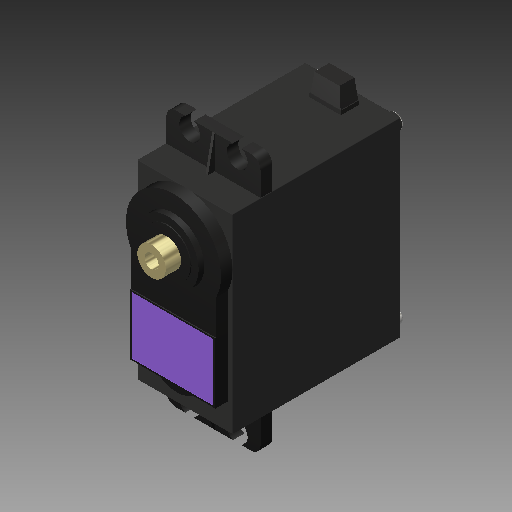
# Autodesk Inventor part: Servomotor
Saved by Autodesk Inventor 2017 (Build 210142000, 142)
## iProperties
Created: 2019-10-22
Part Number: Servomotor
Material: Generic
Document SubType Name: Modeling
Designer: User
Density: 1 g/cm^3
Appearance: Glossy - Black
Mass: 31.6887 g
Surface Area: 70.3531 cm^2
Volume: 31.6887 cm^3
Author: User
Autodesk Inventor part; units mm, degrees
ref_plane "YZ Plane" through (0, 0, 0) normal (1, 0, 0) x (0, 1, 0)
ref_plane "XZ Plane" through (0, 0, 0) normal (0, 1, 0) x (-1, 0, 0)
ref_plane "XY Plane" through (0, 0, 0) normal (0, 0, 1) x (1, 0, 0)
sketch "Sketch1" plane through (0, 0, 0) normal (0, 0, 1) x (1, 0, 0)
  line L0 (-10, 20) -> (10, 20)
  line L1 (10, 20) -> (10, -20)
  line L2 (10, -20) -> (-10, -20)
  line L3 (-10, -20) -> (-10, 20)
  line L4 (-10, 20) -> (10, -20) construction
  line L5 (10, 20) -> (-10, -20) construction
  point P0 (0, 0)
  dimension "d0" = 20
  dimension "d1" = 40
  constraints: 12 end point, 2 midpoint, 2 parallel, 1 horizontal, 1 perpendicular
  measures "d0" distance of L1.end L2.end
  measures "d1" distance of L0.end L1.end
extrude "Extrusion1" add sketch "Sketch1" along normal blind 36.88
chamfer "Chamfer1" distance 1.64 angle 45 4 edges at (-10, 0, 0) (0, 20, 0) (10, 0, 0) (0, -20, 0)
ref_plane "Work Plane1" through (0, 0, 1) normal (0, 0, -1) x (-1, 0, 0)
sketch "Sketch2" plane through (0, 0, 1) normal (0, 0, -1) x (-1, 0, 0)
  line L0 (9.36, -19.36) -> (-9.36, -19.36) projected
  line L1 (-9.36, -19.36) -> (-9.36, 19.36) projected
  line L2 (-9.36, 19.36) -> (9.36, 19.36) projected
  line L3 (9.36, 19.36) -> (9.36, -19.36) projected
  arc A0 (9.36, -15.36) -> (5.36, -19.36) centre (9.36, -19.36) ccw
  point P0 (0, 0)
  dimension "d8" = 8
  constraints: 2 point on circle, 2 point on line, 1 centre point, 1 coincident
  measures "d8" diameter of A0
extrude "Extrusion2" cut sketch "Sketch2" along normal up to next contours L0 A0 L3
mirror "Mirror1" about plane through (0, 0, 0) normal (0, 1, 0) of "Extrusion2"
mirror "Mirror2" about plane through (0, 0, 0) normal (1, 0, 0) of "Extrusion2", "Mirror1"
sketch "Sketch3" plane through (9.36, 19.36, 1) normal (0, 0, -1) x (-1, 0, 0)
  arc A0 (4, -38.72) -> (0, -34.72) centre (0, -38.72) ccw projected
  line L0 (0, -38.72) -> (0, -34.72) projected
  line L1 (4, -38.72) -> (0, -38.72) projected
  line L2 (14.72, -38.72) -> (4, -38.72) projected
  arc A1 (18.72, -34.72) -> (14.72, -38.72) centre (18.72, -38.72) ccw projected
  line L3 (18.72, -4) -> (18.72, -34.72) projected
  arc A2 (14.72, 0) -> (18.72, -4) centre (18.72, 0) ccw projected
  line L4 (4, 0) -> (14.72, 0) projected
  arc A3 (0, -4) -> (4, 0) centre (0, 0) ccw projected
  line L5 (0, -4) -> (0, 0) projected
  line L6 (0, 0) -> (4, 0) projected
  line L7 (0, -34.72) -> (0, -4) projected
  line L8 (18.72, -38.72) -> (14.72, -38.72) projected
  line L9 (18.72, -34.72) -> (18.72, -38.72) projected
  line L10 (18.72, 0) -> (18.72, -4) projected
  line L11 (14.72, 0) -> (18.72, 0) projected
  line L12 (0, -4) -> (0, 0) projected
  line L13 (0, 0) -> (1.6569, 0) construction
  circle A4 centre (1.6569, -1.6569) radius 1.6
  point P0 (9.36, -19.36)
  dimension "d16" = 3.2
  constraints: 2 end point, 1 centre point, 1 horizontal, 1 point on circle
  measures "d16" diameter of A4
extrude "Extrusion4" add sketch "Sketch3" along normal blind 0.8 contours A4
fillet "Fillet1" radius 0.3 1 edges at (9.3031, 17.7031, 0.2)
sketch "Sketch4" plane through (7.7031, 17.7031, 0.2) normal (0, 0, -1) x (-1, 0, 0)
  circle A0 centre (0, 0) radius 1.3 projected
  arc A1 (2.2623, -36.2631) -> (-0.8569, -33.144) centre (-1.6569, -37.0631) ccw projected
  line L0 (-0.8569, -33.144) -> (-0.8569, -2.2623) projected
  arc A2 (-0.8569, -2.2623) -> (2.2623, 0.8569) centre (-1.6569, 1.6569) ccw projected
  line L1 (2.2623, 0.8569) -> (13.144, 0.8569) projected
  arc A3 (13.144, 0.8569) -> (16.2631, -2.2623) centre (17.0631, 1.6569) ccw projected
  line L2 (16.2631, -2.2623) -> (16.2631, -33.144) projected
  arc A4 (16.2631, -33.144) -> (13.144, -36.2631) centre (17.0631, -37.0631) ccw projected
  line L3 (13.144, -36.2631) -> (2.2623, -36.2631) projected
  line L4 (-0.2246, 1.1323) -> (-0.8376, 0.7943)
  line L5 (-0.8376, 0.7943) -> (0.2246, -1.1323)
  line L6 (0.2246, -1.1323) -> (0.8376, -0.7943)
  line L7 (0.8376, -0.7943) -> (-0.2246, 1.1323)
  line L8 (-0.35, -1.1) -> (0.35, 1.1) construction
  line L9 (0.35, -1.1) -> (-0.35, 1.1) construction
  line L10 (-1.1323, -0.2246) -> (-0.7943, -0.8376)
  line L11 (-0.7943, -0.8376) -> (1.1323, 0.2246)
  line L12 (1.1323, 0.2246) -> (0.7943, 0.8376)
  line L13 (0.7943, 0.8376) -> (-1.1323, -0.2246)
  point P0 (7.7031, -17.7031)
  dimension "d21" = 0.7
  dimension "d22" = 2.2
  dimension "d23" = 0.7
  dimension "d24" = 2.2
  constraints: 20 end point, 4 parallel, 2 midpoint, 2 perpendicular
  measures "d21" distance of L6.end L5.end
  measures "d22" distance of L5.end L4.end
  measures "d23" distance of L12.end L12.start
  measures "d24" distance of L12.start L11.start
extrude "Extrusion5" cut sketch "Sketch4" against normal blind 0.5 contours L7 L13 L5 L4 | L13 L12 L11 L7 | L7 L11 L5 L13 | L5 L11 L10 L13 | L7 L6 L5 L11
fillet "Fillet2" radius 0.05 24 edges at (7.0466, 17.2372, 0.2) (7.172, 16.7399, 0.2) (7.6596, 16.8993, 0.2) (8.1691, 17.0466, 0.2) (8.6664, 17.172, 0.2) (8.507, 17.6596, 0.2) (8.3597, 18.1691, 0.2) (8.2343, 18.6664, 0.2) (7.7467, 18.507, 0.2) (7.2372, 18.3597, 0.2) (6.7399, 18.2343, 0.2) (6.8993, 17.7467, 0.2) (6.8993, 17.7467, 0.7) (6.7399, 18.2343, 0.7) (7.0466, 17.2372, 0.7) (7.172, 16.7399, 0.7) (8.1691, 17.0466, 0.7) (7.6596, 16.8993, 0.7) (7.7467, 18.507, 0.7) (7.2372, 18.3597, 0.7) (8.2343, 18.6664, 0.7) (8.3597, 18.1691, 0.7) (8.507, 17.6596, 0.7) (8.6664, 17.172, 0.7)
mirror "Mirror3" about plane through (0, 0, 0) normal (0, 1, 0) of "Extrusion4", "Fillet1", "Extrusion5", "Fillet2"
mirror "Mirror4" about plane through (0, 0, 0) normal (1, 0, 0) of "Extrusion4", "Fillet1", "Extrusion5", "Fillet2", "Mirror3"
sketch "Sketch5" plane through (-10, 20, 36.88) normal (0, 1, 0) x (1, 0, 0)
  line L0 (10, 36.88) -> (17.4, 36.88) construction
  line L1 (13.3, 29.48) -> (6.7, 29.48)
  line L2 (6.7, 29.48) -> (6.7, 33.38)
  line L3 (6.7, 33.38) -> (13.3, 33.38)
  line L4 (13.3, 33.38) -> (13.3, 29.48)
  dimension "d30" = 6.6
  dimension "d31" = 3.9
  constraints: 10 end point, 2 horizontal, 2 parallel, 1 perpendicular
  measures "d30" distance of L2.end L3.end
  measures "d31" distance of L1.end L2.end
extrude "Extrusion6" add sketch "Sketch5" along normal blind 0.8
ref_plane "Work Plane3" through (-10, 24.8, 36.88) normal (0, 1, 0) x (1, 0, 0)
sketch "Sketch6" plane through (-10, 24.8, 36.88) normal (0, 1, 0) x (1, 0, 0)
  line L0 (13.3, 33.38) -> (6.7, 33.38) projected
  line L1 (12.64, 29.87) -> (7.36, 29.87)
  line L2 (7.36, 29.87) -> (7.36, 32.99)
  line L3 (7.36, 32.99) -> (12.64, 32.99)
  line L4 (12.64, 32.99) -> (12.64, 29.87)
  line L5 (13.3, 29.48) -> (6.7, 33.38) construction
  line L6 (6.7, 29.48) -> (13.3, 33.38) construction
  point P0 (10, 36.88)
  point P1 (10, 31.43)
  constraints: 12 end point, 2 midpoint, 2 parallel, 1 horizontal, 1 perpendicular
sketch "Sketch7" plane through (-10, 20.8, 36.88) normal (0, 1, 0) x (1, 0, 0)
  line L0 (13.3, 29.48) -> (6.7, 29.48)
  line L1 (6.7, 29.48) -> (13.3, 29.48) projected
  line L2 (13.135, 33.2825) -> (6.865, 33.2825)
  line L3 (6.865, 33.2825) -> (6.865, 29.5775)
  line L4 (6.865, 29.5775) -> (13.135, 29.5775)
  line L5 (13.135, 29.5775) -> (13.135, 33.2825)
  line L6 (13.3, 33.38) -> (6.7, 29.48) construction
  line L7 (6.7, 33.38) -> (13.3, 29.48) construction
  point P0 (10, 36.88)
  point P1 (10, 31.43)
  constraints: 14 end point, 2 midpoint, 2 parallel, 1 horizontal, 1 perpendicular
loft "Loft1" add profiles "Sketch7", "Sketch6"
sketch "Sketch8" plane through (0, 0, 36.88) normal (0, 0, 1) x (1, 0, 0)
  line L0 (-10, -20) -> (-10, 20) projected
  line L1 (-10, 20) -> (10, 20) projected
  line L2 (10, 20) -> (10, -20) projected
  line L3 (10, -20) -> (-10, -20) projected
  arc A0 (9, 5.6411) -> (-9, 5.6411) centre (0, 10) ccw
  line L4 (0, -14.5) -> (-9, -14.5)
  line L5 (-9, -14.5) -> (-9, 5.6411)
  line L6 (0, -14.5) -> (9, -14.5)
  line L7 (0, -14.5) -> (9, -14.5) construction
  line L8 (9, -14.5) -> (9, 5.6411)
  point P0 (0, 0)
  dimension "d39" = 9
  dimension "d40" = 90
  constraints: 10 end point, 3 tangent, 2 horizontal, 2 point on circle, 1 centre point, 1 collinear, 1 perpendicular
  measures "d39" distance of L4.start L4.end
  measures "d40" angle of L4 L5
extrude "Extrusion7" add sketch "Sketch8" along normal blind 2.4 contours A0 L8 L6 L4 L5
sketch "Sketch9" plane through (0, 0, 39.28) normal (0, 0, 1) x (1, 0, 0)
  line L0 (-9, -14.5) -> (9, -14.5) projected
  line L1 (9, -14.5) -> (9, 5.6411) projected
  line L2 (-9, -14.5) -> (9, -14.5)
  line L3 (9, -14.5) -> (9, -1.74)
  line L4 (9, -1.74) -> (-9, -1.74)
  line L5 (-9, -1.74) -> (-9, -14.5)
  point P0 (0, 0)
  dimension "d46" = 12.76
  constraints: 8 end point, 2 parallel, 1 horizontal, 1 perpendicular, 1 point on line
  measures "d46" distance of L3.end L2.end
extrude "Extrusion8" add sketch "Sketch9" along normal blind 0.2
sketch "Sketch10" plane through (0, 0, 39.48) normal (0, 0, 1) x (1, 0, 0)
  line L0 (-9, -1.74) -> (9, -1.74) projected
  line L1 (9, -1.74) -> (9, -14.5) projected
  line L2 (9, -14.5) -> (-9, -14.5) projected
  line L3 (-9, -14.5) -> (-9, -1.74) projected
  line L4 (9, -14.5) -> (-9, -14.5) projected
  line L5 (-8.55, -14.181) -> (8.55, -14.181)
  line L6 (8.55, -14.181) -> (8.55, -2.059)
  line L7 (8.55, -2.059) -> (-8.55, -2.059)
  line L8 (-8.55, -2.059) -> (-8.55, -14.181)
  point P0 (0, 0)
  constraints: 8 end point, 2 parallel, 1 horizontal, 1 perpendicular
extrude "Extrusion9" cut sketch "Sketch10" against normal blind 0.1 contours L8 L7 L6 L5
sketch "Sketch11" plane through (0, 0, 36.88) normal (0, 0, 1) x (1, 0, 0)
  line L0 (4.5, -14.5) -> (-4.5, -14.5)
  arc A0 (-4.5, -14.5) -> (4.5, -14.5) centre (0, -10.4375) ccw
  point P0 (0, 0)
  constraints: 2 end point, 2 point on circle, 1 centre point, 1 horizontal
extrude "Extrusion10" add sketch "Sketch11" along normal blind 1.7
fillet "Fillet3" radius 0.1 19 edges at (0, -20, 36.88) (10, -5, 36.88) (10, 15, 36.88) (5, 20, 36.88) (-5, 20, 36.88) (-10, 15, 36.88) (-10, -5, 36.88) (-10, 20, 19.26) (-10, -20, 19.26) (10, 20, 19.26) (10, -20, 19.26) (10, 0, 1.64) (8.36, 0, 0) (0, -18.36, 0) (0, -20, 1.64) (-10, 0, 1.64) (-8.36, 0, 0) (0, 18.36, 0) (0, 20, 1.64)
sketch "Sketch12" plane through (0, 0, 39.28) normal (0, 0, 1) x (1, 0, 0)
  line L0 (9, -1.74) -> (9, -14.5)
  circle A0 centre (0, 10) radius 6.5
  dimension "d56" = 13
  constraints: 2 end point, 1 centre point
  measures "d56" diameter of A0
extrude "Extrusion11" add sketch "Sketch12" along normal blind 1.2
sketch "Sketch13" plane through (0, 10, 40.48) normal (0, 0, 1) x (1, 0, 0)
  circle A0 centre (0, 0) radius 6.5 projected
  circle A1 centre (0, 0) radius 5
  point P0 (0, -10)
  dimension "d59" = 10
  constraints: 1 centre point, 1 coincident
  measures "d59" diameter of A1
extrude "Extrusion12" add sketch "Sketch13" along normal blind 0.2 contours A1
sketch "Sketch14" plane through (0, 10, 40.68) normal (0, 0, 1) x (1, 0, 0)
  circle A0 centre (0, 0) radius 6.5 projected
  circle A1 centre (0, 0) radius 3
  point P0 (0, -10)
  dimension "d62" = 6
  constraints: 1 centre point, 1 coincident
  measures "d62" diameter of A1
extrude "Extrusion13" add sketch "Sketch14" along normal blind 3.2 contours A1
sketch "Sketch17" plane through (0, 10, 43.88) normal (0, 0, 1) x (1, 0, 0)
  circle A0 centre (0, 0) radius 1.5
  point P0 (0, -10)
  dimension "d69" = 3
  constraints: 1 centre point
  measures "d69" diameter of A0
extrude "Extrusion15" cut sketch "Sketch17" against normal up to surface (3.2 mm away)
ref_plane "Work Plane4" through (0, 0, 28.48) normal (0, 0, 1) x (1, 0, 0)
sketch "Sketch18" plane through (0, 0, 28.48) normal (0, 0, 1) x (1, 0, 0)
  arc A0 (-10, -19.9) -> (-9.9, -20) centre (-9.9, -19.9) ccw projected
  line L0 (-10, -19.9) -> (-10, 19.9) projected
  arc A1 (-9.9, 20) -> (-10, 19.9) centre (-9.9, 19.9) ccw projected
  line L1 (-9.9, 20) -> (9.9, 20) projected
  arc A2 (10, 19.9) -> (9.9, 20) centre (9.9, 19.9) ccw projected
  line L2 (10, 19.9) -> (10, -19.9) projected
  arc A3 (9.9, -20) -> (10, -19.9) centre (9.9, -19.9) ccw projected
  line L3 (9.9, -20) -> (-9.9, -20) projected
  line L4 (9.9, -20) -> (-9.9, -20)
  line L5 (-9.9, -20) -> (-9.9, -25)
  line L6 (9.9, -25) -> (9.9, -20)
  arc A4 (7.9, -27) -> (9.9, -25) centre (7.9, -25) ccw
  arc A5 (-9.9, -25) -> (-7.9, -27) centre (-7.9, -25) ccw
  arc A6 (5.9165, -27) -> (4.0835, -27) centre (5, -25) ccw
  line L7 (7.9, -27) -> (5.9165, -27)
  arc A7 (-4.0835, -27) -> (-5.9165, -27) centre (-5, -25) ccw
  line L8 (4.0835, -27) -> (-4.0835, -27)
  line L9 (-5.9165, -27) -> (-7.9, -27)
  point P0 (0, 0)
  point P1 (-9.9, -27)
  dimension "d73" = 7
  dimension "d74" = 2
  dimension "d77" = 19.8
  dimension "d78" = 4.4
  constraints: 12 end point, 8 point on circle, 4 centre point, 4 horizontal, 2 tangent, 1 equal radius, 1 parallel, 1 perpendicular, 1 point on line
  measures "d73" distance of point (-9.9, -27) L4.end
  measures "d74" radius of A4
  measures "d77" distance between parallel lines of L5 L6
  measures "d78" diameter of A6
extrude "Extrusion16" add sketch "Sketch18" along normal blind 2.4 contours L3 L6 A4 L7 A6 L8 A7 L9 A5 L5
sketch "Sketch19" plane through (0, 0, 0) normal (1, 0, 0) x (0, 1, 0)
  line L0 (-1.74, 39.48) -> (-1.74, 39.28)
  line L1 (-1.74, 39.28) -> (3.5, 39.28)
  line L2 (3.5, 39.28) -> (3.5, 40.48)
  line L3 (3.5, 40.48) -> (5, 40.48)
  line L4 (5, 40.48) -> (5, 40.68)
  line L5 (5, 40.68) -> (7, 40.68)
  line L6 (7, 40.68) -> (7, 43.88)
  line L7 (7, 43.88) -> (8.5, 43.88)
  line L8 (8.5, 43.88) -> (8.5, 0)
  line L9 (8.5, 0) -> (-18.3186, 0)
  arc A0 (-18.3893, 0.0293) -> (-18.3186, 0) centre (-18.3186, 0.1) ccw
  line L10 (-18.3893, 0.0293) -> (-19.9707, 1.6107)
  arc A1 (-20, 1.6814) -> (-19.9707, 1.6107) centre (-19.9, 1.6814) ccw
  line L11 (-27, 30.88) -> (-20, 30.88)
  arc A2 (-19.9, 36.88) -> (-20, 36.78) centre (-19.9, 36.78) ccw
  line L12 (-19.9, 36.88) -> (-16.5, 36.88)
  line L13 (-16.5, 36.88) -> (-16.5, 38.58)
  line L14 (-16.5, 38.58) -> (-14.5, 38.58)
  line L15 (-14.5, 38.58) -> (-14.5, 39.48)
  line L16 (-14.5, 39.48) -> (-14.181, 39.48)
  line L17 (-14.181, 39.48) -> (-14.181, 39.38)
  line L18 (-14.181, 39.38) -> (-2.059, 39.38)
  line L19 (-2.059, 39.38) -> (-2.059, 39.48)
  line L20 (-2.059, 39.48) -> (-1.74, 39.48)
  line L21 (24.8, 7.01) -> (24.8, 3.89)
  line L22 (24.8, 3.89) -> (20.8, 3.5975)
  line L23 (20.8, 3.5975) -> (20.8, 3.5)
  line L24 (20.8, 3.5) -> (20, 3.5)
  line L25 (20, 3.5) -> (20, 1.6814)
  arc A3 (19.9707, 1.6107) -> (20, 1.6814) centre (19.9, 1.6814) ccw
  line L26 (19.9707, 1.6107) -> (18.3893, 0.0293)
  arc A4 (18.3186, 0) -> (18.3893, 0.0293) centre (18.3186, 0.1) ccw
  line L27 (18.3186, 0) -> (11.5, 0)
  line L28 (11.5, 0) -> (11.5, 43.88)
  line L29 (11.5, 43.88) -> (13, 43.88)
  line L30 (13, 43.88) -> (13, 40.68)
  line L31 (13, 40.68) -> (15, 40.68)
  line L32 (15, 40.68) -> (15, 40.48)
  line L33 (15, 40.48) -> (16.5, 40.48)
  line L34 (16.5, 40.48) -> (16.5, 39.28)
  line L35 (16.5, 39.28) -> (20, 39.28)
  line L36 (20, 39.28) -> (20, 36.88)
  line L37 (20, 36.88) -> (20, 7.4)
  line L38 (20, 7.4) -> (20.8, 7.4)
  line L39 (20.8, 7.4) -> (20.8, 7.3025)
  line L40 (20.8, 7.3025) -> (24.8, 7.01)
  line L41 (-20, 30.88) -> (-20, 32.28)
  line L42 (-20, 32.28) -> (-27, 30.88)
  line L43 (-20, 28.48) -> (-20, 30.88) projected
  line L44 (-20, 30.88) -> (-27, 30.88)
  point P0 (0, 0)
  dimension "d81" = 1.4
  constraints: 88 end point, 10 point on circle, 5 centre point, 1 collinear
  measures "d81" distance of L11.end L41.end
extrude "Extrusion17" add sketch "Sketch19" along normal mid plane 0.5 contours L42 L41 L11
mirror "Mirror5" about plane through (0, 0, 0) normal (0, 1, 0) of "Extrusion17", "Extrusion16"
body "Solid1"
